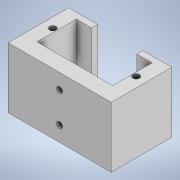
# Autodesk Inventor part: Servo Holder
Saved by Autodesk Inventor 2022 (Build 260153000, 153)
## iProperties
Created: 2023-02-27
Part Number: Servo Holder
Material: Generic
Document SubType Name: Modeling
Designer: zarek
Density: 1 g/cm^3
Appearance: Default
Author: zarek
Autodesk Inventor part; units mm, degrees
ref_plane "YZ Plane" through (0, 0, 0) normal (1, 0, 0) x (0, 1, 0)
ref_plane "XZ Plane" through (0, 0, 0) normal (0, 1, 0) x (-1, 0, 0)
ref_plane "XY Plane" through (0, 0, 0) normal (0, 0, 1) x (1, 0, 0)
sketch "Sketch1" plane through (0, 0, 0) normal (0, 1, 0) x (-1, 0, 0)
  line L0 (0, 0) -> (34, 0)
  line L1 (34, 0) -> (34, -20)
  line L2 (34, -20) -> (0, -20)
  line L3 (0, -20) -> (0, 0)
  dimension "d0" = 34
  dimension "d1" = 20
  constraints: 8 end point, 2 parallel, 1 horizontal, 1 perpendicular
  measures "d0" distance between parallel lines of L3 L1
  measures "d1" distance between parallel lines of L0 L2
extrude "Extrusion1" add sketch "Sketch1" along normal blind 20
sketch "Sketch2" plane through (0, 20, 0) normal (0, 1, 0) x (1, 0, 0)
  line L0 (-29.5, 18) -> (-4.5, 18)
  line L1 (-4.5, 18) -> (-4.5, 5)
  line L2 (-4.5, 5) -> (-29.5, 5)
  line L3 (-29.5, 5) -> (-29.5, 18)
  line L4 (0, 20) -> (-34, 20) projected
  line L5 (-34, 20) -> (-34, 0) projected
  line L6 (-24.5, 20) -> (-9.5, 20)
  line L7 (-9.5, 20) -> (-9.5, 18)
  line L8 (-9.5, 18) -> (-24.5, 18)
  line L9 (-24.5, 18) -> (-24.5, 20)
  line L10 (0, 0) -> (0, 20) projected
  point P0 (-9.5, 20)
  dimension "d6" = 25
  dimension "d7" = 13
  dimension "d8" = 2
  dimension "d9" = 4.5
  dimension "d12" = 5
  dimension "d13" = 5
  dimension "d26" = 4.5
  constraints: 16 end point, 4 parallel, 2 horizontal, 2 perpendicular, 2 point on line
  measures "d6" distance between parallel lines of L1 L3
  measures "d7" distance between parallel lines of L2 L0
  measures "d8" distance between parallel lines of L0 L4
  measures "d9" distance between parallel lines of L3 L5
  measures "d12" distance between parallel lines of L7 L1
  measures "d13" distance between parallel lines of L3 L9
  measures "d26" distance between parallel lines of L10 L1
extrude "Extrusion2" cut sketch "Sketch2" against normal blind 33
sketch "Sketch3" plane through (-4.5, 20, -5) normal (0, 0, -1) x (-1, 0, 0)
  line L0 (29.5, -20) -> (29.5, 0) projected
  line L1 (-4.5, -20) -> (-4.5, 0) projected
  line L2 (29.5, 0) -> (-4.5, 0) projected
  line L3 (12.5, 0) -> (12.5, -20)
  circle A0 centre (12.5, -5) radius 1
  circle A1 centre (12.5, -15) radius 1
  dimension "d27" = 2
  dimension "d28" = 2
  dimension "d29" = 5
  dimension "d30" = 5
  dimension "d33" = 10
  constraints: 2 centre point, 2 end point, 2 point on line, 1 midpoint, 1 vertical
  measures "d27" diameter of A0
  measures "d28" diameter of A1
  measures "d29" distance of A0.centre L3.start
  measures "d30" distance of L3.end A1.centre
  measures "d33" distance of A1.centre A0.centre
extrude "Extrusion3" cut sketch "Sketch3" against normal through all
sketch "Sketch4" plane through (0, 20, 0) normal (0, 1, 0) x (1, 0, 0)
  line L0 (-34, 20) -> (-34, 0) projected
  line L1 (-29.5, 18) -> (-29.5, 5) projected
  line L2 (-9.5, 18) -> (-4.5, 18) projected
  line L3 (-29.5, 5) -> (-4.5, 5)
  line L4 (-4.5, 5) -> (-4.5, 18)
  line L5 (-4.5, 18) -> (-29.5, 18)
  line L6 (-29.5, 18) -> (-29.5, 5)
  line L7 (-29.5, 11.5) -> (-34, 11.5)
  line L8 (-29.5, 11.5) -> (0, 11.5)
  line L9 (0, 0) -> (0, 20) projected
  circle A0 centre (-3.25, 11.5) radius 0.8
  circle A1 centre (-30.75, 11.5) radius 0.8
  dimension "d21" = 1.6
  dimension "d22" = 3.25
  dimension "d31" = 1.6
  dimension "d32" = 3.25
  constraints: 12 end point, 5 point on line, 2 centre point, 2 parallel, 2 perpendicular, 1 horizontal, 1 midpoint
  measures "d21" diameter of A0
  measures "d22" distance of L8.end A0.centre
  measures "d31" diameter of A1
  measures "d32" distance of L7.end A1.centre
hole "Hole1" at (-30.75, 20, -11.5) at (-3.25, 20, -11.5) direction (0, -1, 0) diameter 2.1211 depth 7.1 tip angle 118 countersink diameter 2.159 countersink angle 82 thread size "M2.5x0.35" class "6H" standard "ANSI Metric M Profile"
sketch "Sketch6" plane through (-4.5, 20, -5) normal (0, 0, -1) x (-1, 0, 0)
  line L0 (29.5, -20) -> (29.5, 0)
  line L1 (-4.5, -20) -> (-4.5, 0)
  line L2 (29.5, 0) -> (-4.5, 0)
  line L3 (12.5, 0) -> (12.5, -20)
  circle A0 centre (12.5, -5) radius 1
  circle A1 centre (12.5, -15) radius 1
  circle A2 centre (12.5, -5) radius 1 projected
  circle A3 centre (12.5, -5) radius 3.5
  circle A4 centre (12.5, -15) radius 3.5
  dimension "d41" = 2
  dimension "d42" = 2
  dimension "d43" = 5
  dimension "d44" = 5
  dimension "d45" = 10
  dimension "d46" = 7
  dimension "d47" = 7
  constraints: 8 end point, 4 centre point, 2 coincident, 2 point on line, 1 midpoint, 1 vertical
  measures "d41" diameter of A0
  measures "d42" diameter of A1
  measures "d43" distance of A0.centre L3.start
  measures "d44" distance of L3.end A1.centre
  measures "d45" distance of A1.centre A0.centre
  measures "d46" diameter of A3
  measures "d47" diameter of A4
extrude "Extrusion5" cut sketch "Sketch6" against normal blind 2 contours A3 L3 A0 | A4 L3 A1 | L3 A1 A4 | L3 A0 A3
body "Solid1"
